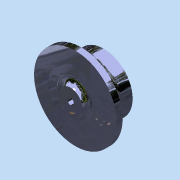
# Autodesk Inventor part: Bauteil1
Saved by Autodesk Inventor 2018 (Build 220112000, 112)
## iProperties
Created: 2014-12-29
Part Number: Bauteil1
Document SubType Name: Modeling
Designer: Marcel
Density: 1 g/cm^3
Material: Allgemein
Appearance: Chrom - poliert - blau
Author: Marcel
Autodesk Inventor part; units mm, degrees
ref_plane "YZ Plane" through (0, 0, 0) normal (1, 0, 0) x (0, 1, 0)
ref_plane "XZ Plane" through (0, 0, 0) normal (0, 1, 0) x (-1, 0, 0)
ref_plane "XY Plane" through (0, 0, 0) normal (0, 0, 1) x (1, 0, 0)
sketch "Skizze5" plane through (0, 0, 0) normal (0, 0, 1) x (1, 0, 0)
  line L0 (0, 0) -> (14.5, 0)
  line L1 (33.3, 6) -> (50.9, 6)
  line L2 (33.3, 6) -> (23, 5.6403)
  arc A0 (23, 5.6403) -> (14.5, 0) centre (23.34, -4.0971) ccw
  line L3 (50.9, 6) -> (50.9, 7.3)
  line L4 (50.9, 7.3) -> (50.88, 7.3)
  line L5 (50.88, 7.3) -> (50.88, 13.3)
  line L6 (0, 0) -> (9.7, 0)
  line L7 (9.7, 0) -> (9.7, 48)
  line L8 (9.7, 48) -> (0, 48)
  line L9 (0, 48) -> (0, 0)
  line L10 (9.7, 48) -> (9.7, 41)
  line L11 (9.7, 41) -> (35.5, 41)
  line L12 (35.5, 41) -> (35.5, 17.4211)
  line L13 (50.88, 13.3) -> (35.5, 17.4211)
  arc A1 (35.5, 28.1636) -> (45.8765, 14.6407) centre (49.5, 28.1636) ccw
  line L14 (50.88, 13.3) -> (35.0608, 13.3)
  dimension "d21" = 14.5
  dimension "d22" = 50.9
  dimension "d23" = 6
  dimension "d24" = 33.3
  dimension "d25" = 23
  dimension "d26" = 2
  dimension "d28" = 1.3
  dimension "d29" = 0.02
  dimension "d30" = 6
  dimension "d31" = 9.7
  dimension "d32" = 48
  dimension "d33" = 7
  dimension "d47" = 25.8
  dimension "d48" = 35.5
  dimension "d49" = 105
  dimension "d53" = 14
  dimension "d54" = 15
  dimension "d55" = 35
  constraints: 31 end point, 8 perpendicular, 4 point on circle, 4 point on line, 3 tangent, 2 centre point, 2 horizontal, 1 parallel
  measures "d21" distance of L0.start L0.end
  measures "d22" horizontal distance of L1.end L0.start
  measures "d23" distance between parallel lines of L1 L0
  measures "d24" horizontal distance of L1.start L0.start
  measures "d25" horizontal distance of L0.start L2.end
  measures "d26" angle of L1 L2
  measures "d28" distance of L1.end L3.end
  measures "d29" distance of L3.end L4.end
  measures "d30" distance of L4.end L5.end
  measures "d31" distance of L0.start L6.end
  measures "d32" distance of L6.end L7.end
  measures "d33" distance of L7.end L10.end
  measures "d47" distance of L10.end L11.end
  measures "d48" distance between parallel lines of L12 L9
  measures "d49" angle of L13 L5
  measures "d53" radius of A1
  measures "d54" angle of L14 L13
  measures "d55" distance between parallel lines of L1 L11
revolve "Umdrehung1" add sketch "Skizze5" angle 360 about axis through (0, 48, 0) along (0, -1, 0)
sketch "Skizze6" plane through (0, 0, 0) normal (0, -1, 0) x (1, 0, 0)
  circle A0 centre (0, 0) radius 14.5 projected
hole "Hole2" at (0, 0, 0) direction (0, 1, 0) diameter 8 end through all
